extractor connector (Autodesk Fusion 360 design; units mm, degrees)
Autodesk Fusion 360 part; units mm, degrees
sketch "Sketch1" plane through (0, 0, 0) normal (0, 1, 0) x (1, 0, 0)
  circle A0 centre (0, 0) radius 63.5
  circle A1 centre (0, 0) radius 68.5
  dimension "d1" = 127
  dimension "d2" = 137
  constraint coincident A0.centre A1.centre
  constraint concentric A0 A1
  measures "d1" diameter of A0
  measures "d2" diameter of A1
extrude "Extrude1" add sketch "Sketch1" along normal blind 30 makes body 1
copy_body "CutPasteBodies1" bodies 1 removing the originals makes body 2 in component "Component"
sketch "Sketch1 (2)" plane through (0, 30, 0) normal (0, 1, 0) x (-1, 0, 0) in component "Component"
  circle A0 centre (0, 0) radius 63.5
  circle A1 centre (0, 0) radius 68.5
  line L0 (60, -60) -> (-60, -60)
  line L1 (-60, -60) -> (-60, 60)
  line L2 (-60, 60) -> (60, 60)
  line L3 (60, 60) -> (60, -60)
  line L4 (60, -60) -> (-60, 60) construction
  line L5 (-60, -60) -> (60, 60) construction
  dimension "d7" = 120
  dimension "d8" = 120
  constraint perpendicular L0 L1
  constraint parallel L0 L2
  constraint parallel L1 L3
  constraint horizontal L0
  constraint coincident L4 A0.centre
  constraint coincident L5 A0.centre
  constraint coincident A0.centre A1.centre
  measures "d7" distance of L0.end L1.end
  measures "d8" distance of L1.end L2.end
extrude "Extrude1'" add sketch "Sketch1 (2)" along normal blind 40 contours A0 L3 | A0 A1 L3 | A0 A1 L2 L3 | A0 A1 L0 L3 | A0 L2 | A0 A1 L2 | A1 L2 L3 | A0 A1 L0 | A0 L0 | A1 L0 L3 | A0 A1 L1 L2 | A0 A1 L0 L1 | A0 L1 | A0 A1 L1 | A1 L1 L2 | A1 L0 L1 bodies 2 in component "Component"
delete_face "DeleteFace1" 1 faces at (6.9302, 43.3333, 60) on bodies 2 in component "Component"
delete_face "DeleteFace2" 1 faces at (-60, 56.6667, 6.9302) on bodies 2 in component "Component"
delete_face "DeleteFace3" 1 faces at (-6.9302, 43.3333, -60) on bodies 2 in component "Component"
delete_face "DeleteFace4" 1 faces at (60, 43.3333, -6.9302) on bodies 2 in component "Component"
sketch "Sketch2" plane through (0, 70, 0) normal (0, 1, 0) x (-1, 0, 0) in component "Component"
  circle A0 centre (0, 0) radius 63.5
  arc A1 (33.0492, 60) -> (-33.0492, 60) centre (0, 0) ccw
  line L0 (-33.0492, 60) -> (-60, 60)
  line L1 (-60, 60) -> (-60, 33.0492)
  arc A2 (-60, 33.0492) -> (-60, -33.0492) centre (0, 0) ccw
  line L2 (-60, -33.0492) -> (-60, -60)
  line L3 (-60, -60) -> (-33.0492, -60)
  arc A3 (-33.0492, -60) -> (33.0492, -60) centre (0, 0) ccw
  line L4 (33.0492, -60) -> (60, -60)
  line L5 (60, -60) -> (60, -33.0492)
  arc A4 (60, -33.0492) -> (60, 33.0492) centre (0, 0) ccw
  line L6 (60, 33.0492) -> (60, 60)
  line L7 (60, 60) -> (33.0492, 60)
  line L8 (60, 60) -> (-60, 60)
  line L9 (-60, 60) -> (-60, -60)
  line L10 (-60, -60) -> (60, -60)
  line L11 (60, -60) -> (60, 60)
  constraint horizontal L8
  constraint vertical L9
  constraint horizontal L10
  constraint vertical L11
  constraint coincident L2.end L3.start
  constraint coincident L6.end L7.start
extrude "Extrude2" cut sketch "Sketch2" against normal blind 20 contours A0 A4 L11 | A0 A1 L8 | A0 A3 L10 | A0 A2 L9 bodies 2 in component "Component"
sketch "Sketch3" plane through (0, 70, 0) normal (0, 1, 0) x (-1, 0, 0) in component "Component"
  line L0 (-20.7906, 60) -> (-60, 60)
  line L1 (-60, 60) -> (-60, 20.7906)
  arc A0 (-20.7906, 60) -> (-60, 20.7906) centre (0, 0) ccw
  line L2 (-60, 60) -> (60, 60)
  line L3 (60, 60) -> (60, -60)
  line L4 (60, -60) -> (-60, -60)
  line L5 (-60, -60) -> (-60, 60)
  line L6 (-60, 60) -> (60, -60) construction
  line L7 (60, 60) -> (-60, -60) construction
  dimension "d13" = 120
  dimension "d14" = 120
  constraint perpendicular L2 L3
  constraint parallel L2 L4
  constraint parallel L3 L5
  constraint horizontal L2
  constraint coincident L6 A0.centre
  constraint coincident L7 A0.centre
  constraint coincident A0.centre origin
  measures "d13" distance of L3.end L4.end
  measures "d14" distance of L2.end L3.end
component "Component" placed x (1, 0, 0) y (0, 1, 0) z (0, 0, 1) at (0, 0, 0)
